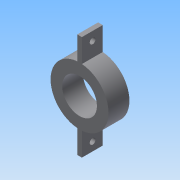
# Autodesk Inventor part: torchHolder
Saved by Autodesk Inventor 2015 (Build 190159000, 159)
## iProperties
Created: 2014-09-02
Part Number: torchHolder
Material: Generic
Document SubType Name: Modeling
Designer: shohei
Density: 1 g/cm^3
Appearance: Default
Author: shohei
Autodesk Inventor part; units mm, degrees
ref_plane "YZ Plane" through (0, 0, 0) normal (1, 0, 0) x (0, 1, 0)
ref_plane "XZ Plane" through (0, 0, 0) normal (0, 1, 0) x (-1, 0, 0)
ref_plane "XY Plane" through (0, 0, 0) normal (0, 0, 1) x (1, 0, 0)
sketch "Sketch4" plane through (0, 0, 0) normal (0, 1, 0) x (-1, 0, 0)
  line L0 (34.9719, 0) -> (-34.9719, 0) projected
  line L1 (0, -63) -> (0, 63) projected
  line L2 (0, -63) -> (0, 63) projected
  circle A0 centre (0, 0) radius 15
  line L3 (2, 24.8997) -> (2, 45)
  line L4 (2, 45) -> (0, 45)
  line L5 (2, -24.8997) -> (2, -45)
  line L6 (2, -45) -> (0, -45)
  line L7 (-2, 24.8997) -> (-2, 45)
  line L8 (-2, 45) -> (0, 45)
  line L9 (-2, -24.8997) -> (-2, -45)
  line L10 (-2, -45) -> (0, -45)
  arc A1 (-2, 24.8997) -> (-2, -24.8997) centre (0, 0) ccw
  arc A2 (2, -24.8997) -> (2, 24.8997) centre (0, 0) ccw
  dimension "d42" = 30
  dimension "d44" = 2
  dimension "d45" = 45
  constraints: 16 end point, 7 symmetric about line, 4 point on circle, 3 centre point, 2 coincident, 1 perpendicular, 1 point on line, 1 vertical
  measures "d42" diameter of A0
  measures "d44" distance of L3.end L4.end
  measures "d45" distance between parallel lines of L0 L4
extrude "Extrusion6" add sketch "Sketch4" along normal blind 18 contours A2 L5 L6 L1 A0 L0 | L0 A0 L1 L4 L3 A2 | A0 L0 A1 L7 L8 L1 | L1 L10 L9 A1 L0 A0
sketch "Sketch5" plane through (-2, 0, -45) normal (-1, 0, 0) x (0, 0, 1)
  circle A0 centre (82.5, 9.257) radius 2.5
  circle A1 centre (7.5, 9.257) radius 2.5
  line L0 (0, 0) -> (0, 18) projected
  line L1 (45, -3.6) -> (45, 21.6) projected
  line L2 (-18, 0) -> (108, 0) projected
  point P0 (45, 0)
  dimension "d48" = 5
  dimension "d49" = 5
  dimension "d50" = 75
  dimension "d52" = 37.5
  constraints: 2 centre point
  measures "d48" diameter of A0
  measures "d49" diameter of A1
  measures "d50" distance of A1.centre A0.centre
  measures "d52" distance from line of L1 A0.centre
extrude "Extrusion7" cut sketch "Sketch5" against normal through all
body "Solid4"
